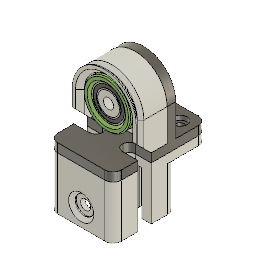
idler-pulley (Autodesk Fusion 360 design; units mm, degrees)
Autodesk Fusion 360 part; units mm, degrees
sketch "Sketch1" plane through (0, 0, 0) normal (0, 0, 1) x (1, 0, 0)
  circle A0 centre (0, 0) radius 7.65
  circle A1 centre (0, 0) radius 10.5
  circle A2 centre (0, 0) radius 9.15
  dimension "d871" = 15.3
  dimension "d873" = 1.5
  dimension "d888" = 0
  dimension "d889" = 0
  dimension "d890" = 0
  dimension "d891" = 0
  dimension "d901" = 21
  constraint coincident A0.centre A1.centre
  constraint concentric A0 A1
  measures "d871" diameter of A0
  measures "d901" diameter of A1
extrude "Extrude1" add sketch "Sketch1" along normal blind 4 contours A1 | A2 makes body 1
sketch "Sketch2" plane through (0, 0, 0) normal (0, 1, 0) x (1, 0, 0)
  line L0 (-10.5, -4) -> (10.5, -4)
  line L1 (-10.5, 0) -> (10.5, 0)
  line L2 (10.5, -4) -> (10.5, -3.5)
  line L3 (10.5, -3.5) -> (9, -2)
  line L4 (9, -2) -> (10.5, -0.5)
  line L5 (10.5, -0.5) -> (10.5, 0)
  line L6 (0, 0) -> (0, -4)
  line L7 (7.65, -4) -> (-7.65, -4)
  line L8 (7.65, -4) -> (7.65, 0)
  line L9 (10.5, -0.5) -> (10.5, -3.5)
  line L10 (9, -2) -> (10.5, -2) construction
  dimension "d882" = 1.5
  dimension "d885" = 0.5
  constraint coincident L0.end L2.start
  constraint perpendicular L0 L2
  constraint coincident L1.end L5.end
  constraint vertical L5
  constraint perpendicular L3 L4
  constraint coincident L6.start origin
  constraint perpendicular L1 L6
  constraint coincident L7.start L8.start
  constraint coincident L1 L8.end
  constraint perpendicular L1 L8
  constraint midpoint L9 L10.end
  constraint horizontal L10
  measures "d882" horizontal distance of L2.end L3.end
  measures "d885" distance of L0.end L2.end
revolve "Revolve1" cut sketch "Sketch2" angle 360 about axis through (0, 0, 0) along (0, 0, 1) contours L3 L4 L9 bodies 1
fillet "Fillet1" radius 1 1 edges at (-8.3909, -3.2545, 2) on bodies 1
ref_plane "WorkPlane1" through (0, 0, 610) normal (0, 0, 1) x (1, 0, 0) in component "top cap"
sketch "Sketch1 (2)" plane through (0, 0, 610) normal (0, 0, 1) x (1, 0, 0) in component "top cap"
  line L0 (14.5, 28.2) -> (-14.5, 28.2)
  line L1 (-14.5, 28.2) -> (-14.5, -14.2)
  line L2 (-14.5, -14.2) -> (14.5, -14.2)
  line L3 (14.5, -14.2) -> (14.5, 28.2)
  line L4 (14.5, 0) -> (-14.5, 0) construction
  circle A0 centre (0, 0) radius 2.5
  arc A1 (3.213, -4.7686) -> (2.0816, -4.3) centre (2.0816, -5.9) ccw
  line L5 (-2.0816, -4.3) -> (2.0816, -4.3)
  arc A2 (-2.0816, -4.3) -> (-3.213, -4.7686) centre (-2.0816, -5.9) ccw
  line L6 (-5.2007, -6.7563) -> (-3.213, -4.7686)
  arc A3 (-5.2007, -6.7563) -> (-5.23, -6.8271) centre (-5.13, -6.8271) ccw
  line L7 (-5.23, -7.7) -> (-5.23, -6.8271)
  arc A4 (-5.23, -7.7) -> (-5.13, -7.8) centre (-5.13, -7.7) ccw
  line L8 (-3.6, -7.8) -> (-5.13, -7.8)
  arc A5 (-2.7, -8.7) -> (-3.6, -7.8) centre (-3.6, -8.7) ccw
  line L9 (-2.7, -9) -> (-2.7, -8.7)
  line L10 (-2.7, 8.7) -> (-2.7, 9)
  arc A6 (-3.6, 7.8) -> (-2.7, 8.7) centre (-3.6, 8.7) ccw
  line L11 (-5.13, 7.8) -> (-3.6, 7.8)
  arc A7 (-5.13, 7.8) -> (-5.23, 7.7) centre (-5.13, 7.7) ccw
  line L12 (-5.23, 6.8271) -> (-5.23, 7.7)
  arc A8 (-5.23, 6.8271) -> (-5.2007, 6.7563) centre (-5.13, 6.8271) ccw
  line L13 (-3.213, 4.7686) -> (-5.2007, 6.7563)
  arc A9 (-3.213, 4.7686) -> (-2.0816, 4.3) centre (-2.0816, 5.9) ccw
  line L14 (2.0816, 4.3) -> (-2.0816, 4.3)
  arc A10 (2.0816, 4.3) -> (3.213, 4.7686) centre (2.0816, 5.9) ccw
  line L15 (5.2007, 6.7563) -> (3.213, 4.7686)
  arc A11 (5.2007, 6.7563) -> (5.23, 6.8271) centre (5.13, 6.8271) ccw
  line L16 (5.23, 7.7) -> (5.23, 6.8271)
  arc A12 (5.23, 7.7) -> (5.13, 7.8) centre (5.13, 7.7) ccw
  line L17 (3.6, 7.8) -> (5.13, 7.8)
  arc A13 (2.7, 8.7) -> (3.6, 7.8) centre (3.6, 8.7) ccw
  line L18 (2.7, 9) -> (2.7, 8.7)
  line L19 (2.7, -8.7) -> (2.7, -9)
  arc A14 (3.6, -7.8) -> (2.7, -8.7) centre (3.6, -8.7) ccw
  line L20 (5.13, -7.8) -> (3.6, -7.8)
  arc A15 (5.13, -7.8) -> (5.23, -7.7) centre (5.13, -7.7) ccw
  line L21 (5.23, -6.8271) -> (5.23, -7.7)
  arc A16 (5.23, -6.8271) -> (5.2007, -6.7563) centre (5.13, -6.8271) ccw
  line L22 (3.213, -4.7686) -> (5.2007, -6.7563)
  line L23 (10.2, 10.2) -> (-10.2, 10.2)
  line L24 (-10.2, 10.2) -> (-10.2, -10.2)
  line L25 (-10.2, -10.2) -> (10.2, -10.2)
  line L26 (10.2, -10.2) -> (10.2, 10.2)
  line L27 (-2.7, -9) -> (-2.7, -10.2)
  line L28 (2.7, -9) -> (2.7, -10.2)
  line L29 (-2.7, 9) -> (-2.7, 10.2)
  line L30 (2.7, 9) -> (2.7, 10.2)
  line L31 (14.5, 3) -> (4.5, 3)
  line L32 (4.5, 3) -> (4.5, -3)
  line L33 (4.5, -3) -> (14.5, -3)
  line L34 (14.5, -3) -> (14.5, 3)
  line L35 (-14.5, 3) -> (-4.5, 3)
  line L36 (-4.5, 3) -> (-4.5, -3)
  line L37 (-4.5, -3) -> (-14.5, -3)
  line L38 (-14.5, -3) -> (-14.5, 3)
  line L39 (14.5, 14.2) -> (-14.5, 14.2)
  dimension "d1200" = 10.2
  dimension "d1201" = 10.2
  dimension "d1202" = 10.2
  dimension "d1203" = 10.2
  dimension "d1227" = 6
  dimension "d1228" = 10
  dimension "d1229" = 10
  dimension "d1230" = 6
  dimension "d1239" = 4
  dimension "d1240" = 14
  dimension "d1241" = 29
  constraint horizontal L0
  constraint vertical L1
  constraint horizontal L2
  constraint vertical L3
  constraint midpoint A0.centre L4
  constraint tangent L21 A16
  constraint tangent A15 L21
  constraint tangent L20 A15
  constraint tangent L17 A13
  constraint tangent L6 A3
  constraint tangent A14 L20
  constraint tangent A4 L8
  constraint tangent A13 L18
  constraint tangent L15 A11
  constraint tangent A10 L15
  constraint tangent L14 A10
  constraint tangent L13 A9
  constraint tangent A8 L13
  constraint tangent L8 A5
  constraint tangent L12 A8
  constraint tangent A9 L14
  constraint tangent L11 A7
  constraint tangent L10 A6
  constraint tangent L5 A2
  constraint tangent A6 L11
  constraint tangent A1 L22
  constraint tangent A12 L17
  constraint tangent L16 A12
  constraint tangent A16 L22
  constraint tangent A11 L16
  constraint tangent A5 L9
  constraint tangent A3 L7
  constraint tangent L19 A14
  constraint tangent A2 L6
  constraint tangent L7 A4
  constraint tangent A7 L12
  constraint tangent A1 L5
  constraint coincident L25 L27.end
  constraint perpendicular L25 L27
  constraint coincident L25 L28.end
  constraint perpendicular L25 L28
  constraint coincident L23 L29.end
  constraint perpendicular L23 L29
  constraint coincident L23 L30.end
  constraint perpendicular L23 L30
  constraint parallel L0 L23
  constraint parallel L1 L24
  constraint parallel L2 L25
  constraint parallel L3 L26
  constraint horizontal L31
  constraint vertical L32
  constraint horizontal L33
  constraint vertical L34
  constraint horizontal L35
  constraint vertical L36
  constraint horizontal L37
  constraint vertical L38
  constraint coincident L3 L39.start
  constraint coincident L1 L39.end
  constraint perpendicular L1 L39
  constraint coincident L1 L4.end
  constraint coincident L3 L4.start
  measures "d1200" distance of A0.centre L26
  measures "d1201" distance of L4 L25
  measures "d1202" distance of A0.centre L24
  measures "d1203" distance of A0.centre L23
  measures "d1227" distance of L31.end L32.end
  measures "d1228" distance of L31.start L31.end
  measures "d1229" distance of L36.end L37.end
  measures "d1230" distance of L35.start L37.end
  measures "d1239" distance of L23 L39
  measures "d1240" distance of L0 L39
  measures "d1241" distance of L1.end L2.end
extrude "Extrude1'" add sketch "Sketch1 (2)" along normal blind 4 separate body contours L0 L1 L3 L39 | L1 L3 L23 L24 L26 L31 L35 L39 | L1 L2 L3 L24 L25 L26 L33 L37 | A1 L5 A2 L6 A3 L7 A4 L8 A5 L9 L10 A6 L11 A7 L12 A8 L13 A9 L14 A10 L15 A11 L16 A12 L17 A13 L18 L19 A14 L20 A15 L21 A16 L22 L23 L24 L25 L26 L27 L28 L29 L30 L31 L32 L33 L35 L36 L37 | L10 A6 L11 A7 L12 A8 L13 A9 L14 A10 L15 A11 L16 A12 L17 A13 L18 L23 L29 L30 | A1 L5 A2 L6 A3 L7 A4 L8 A5 L9 L19 A14 L20 A15 L21 A16 L22 L25 L27 L28 | A0 makes body 2 in component "top cap"
extrude "Extrude2" add sketch "Sketch1 (2)" against normal blind 20 contours L1 L3 L23 L24 L26 L31 L35 L39 | L1 L2 L3 L24 L25 L26 L33 L37 | L10 A6 L11 A7 L12 A8 L13 A9 L14 A10 L15 A11 L16 A12 L17 A13 L18 L23 L29 L30 bodies 2 in component "top cap"
fillet "Fillet1'" radius 1.5 4 edges at (10.2, 10.2, 600) (-10.2, 10.2, 600) (-10.2, -10.2, 600) (10.2, -10.2, 600) on bodies 2 in component "top cap"
fillet "Fillet1'" radius 3.75 6 edges at (-14.5, -14.2, 602) (14.5, -14.2, 602) (-14.5, 28.2, 612) (14.5, 28.2, 612) (-14.5, 14.2, 600) (14.5, 14.2, 600) on bodies 2 in component "top cap"
fillet "Fillet2" radius 3 4 edges at (4.5, -3, 612) (4.5, 3, 612) (-4.5, 3, 612) (-4.5, -3, 612) on bodies 2 in component "top cap"
sketch "Sketch3" plane through (0, 0, 614) normal (0, 0, 1) x (-1, 0, 0) in component "top cap"
  arc A0 (-10.75, 14.2) -> (-14.5, 10.45) centre (-10.75, 10.45) ccw
  line L0 (-14.5, 10.45) -> (-14.5, 3)
  line L1 (-10.75, -28.2) -> (10.75, -28.2)
  line L2 (14.5, -24.45) -> (14.5, -3)
  arc A1 (14.5, 10.45) -> (10.75, 14.2) centre (10.75, 10.45) ccw
  line L3 (10.75, 14.2) -> (-10.75, 14.2)
  line L4 (-14.5, 3) -> (-7.5, 3)
  arc A2 (-7.5, -3) -> (-7.5, 3) centre (-7.5, 0) ccw
  line L5 (-7.5, -3) -> (-14.5, -3)
  line L6 (-14.5, -3) -> (-14.5, -24.45)
  line L7 (14.5, -3) -> (7.5, -3)
  arc A3 (7.5, 3) -> (7.5, -3) centre (7.5, 0) ccw
  line L8 (7.5, 3) -> (14.5, 3)
  line L9 (14.5, 3) -> (14.5, 10.45)
  line L10 (0, -28.2) -> (0, 14.2) construction
  arc A4 (-14.5, -24.45) -> (-10.75, -28.2) centre (-10.75, -24.45) ccw
  arc A5 (10.75, -28.2) -> (14.5, -24.45) centre (10.75, -24.45) ccw
  circle A6 centre (-8.5, -22.2) radius 2.3
  circle A7 centre (8.5, -22.2) radius 2.3
  dimension "d1243" = 4.6
  dimension "d67" = 6
  dimension "d68" = 6
  constraint midpoint L1 L10.start
  constraint midpoint L3 L10.end
  constraint symmetric L10 A6 A7
  measures "d1243" diameter of A6
  measures "d67" distance of L1 A6.centre
  measures "d68" distance of L6 A6.centre
extrude "Extrude4" cut sketch "Sketch3" against normal up to surface (4 mm away) contours A6 | A7 bodies 2 in component "top cap"
sketch "Sketch4" plane through (0, -14.2, 0) normal (0, -1, 0) x (1, 0, 0) in component "top cap"
  line L0 (10.75, 590) -> (10.75, 614)
  line L1 (10.75, 614) -> (-10.75, 614)
  line L2 (-10.75, 614) -> (-10.75, 590)
  line L3 (-10.75, 590) -> (10.75, 590)
  circle A0 centre (0, 598) radius 2.25
  circle A1 centre (0, 598) radius 4.2
  dimension "d1305" = 4.5
  dimension "d1306" = 8.4
  constraint concentric A0 A1
  measures "d1305" diameter of A0
  measures "d1306" diameter of A1
extrude "Extrude7" cut sketch "Sketch4" against normal up to surface (4 mm away) contours A0 bodies 2 in component "top cap"
extrude "Extrude8" cut sketch "Sketch4" against normal blind 2 contours A1 bodies 2 in component "top cap"
chamfer "Chamfer2" distance 1.5 angle 45 1 edges at (-3.9158, -14.2, 599.5188) on bodies 2 in component "top cap"
ref_plane "WorkPlane1" through (0, 0, 612) normal (0, 0, 1) x (1, 0, 0) in component "top adapter"
sketch "Sketch1 (3)" plane through (0, 0, 614) normal (0, 0, 1) x (1, 0, 0) in component "top adapter"
  line L0 (-14.5, 14.2) -> (14.5, 14.2)
  line L1 (14.5, 14.2) -> (14.5, 10.2)
  line L2 (14.5, 10.2) -> (-14.5, 10.2)
  line L3 (-14.5, 10.2) -> (-14.5, 14.2)
  circle A0 centre (8.5, 22.2) radius 2.3
  circle A1 centre (-8.5, 22.2) radius 2.3
  arc A2 (14.5, 24.45) -> (10.75, 28.2) centre (10.75, 24.45) ccw
  line L4 (10.75, 28.2) -> (-10.75, 28.2)
  arc A3 (-10.75, 28.2) -> (-14.5, 24.45) centre (-10.75, 24.45) ccw
  line L5 (-14.5, 24.45) -> (-14.5, 3)
  line L6 (-14.5, 3) -> (-7.5, 3)
  arc A4 (-7.5, -3) -> (-7.5, 3) centre (-7.5, 0) ccw
  line L7 (-7.5, -3) -> (-14.5, -3)
  line L8 (-14.5, -3) -> (-14.5, -10.45)
  arc A5 (-14.5, -10.45) -> (-10.75, -14.2) centre (-10.75, -10.45) ccw
  line L9 (-10.75, -14.2) -> (10.75, -14.2)
  arc A6 (10.75, -14.2) -> (14.5, -10.45) centre (10.75, -10.45) ccw
  line L10 (14.5, -10.45) -> (14.5, -3)
  line L11 (14.5, -3) -> (7.5, -3)
  arc A7 (7.5, 3) -> (7.5, -3) centre (7.5, 0) ccw
  line L12 (7.5, 3) -> (14.5, 3)
  line L13 (14.5, 3) -> (14.5, 24.45)
  line L14 (0, 14.2) -> (0, 28.2) construction
  circle A8 centre (8.5, 22.2) radius 3.1
  circle A9 centre (-8.5, 22.2) radius 3.1
  circle A10 centre (8.5, 22.2) radius 1.75
  circle A11 centre (-8.5, 22.2) radius 1.75
  point P0 (10.75, 24.45)
  point P1 (10.75, 24.45)
  dimension "d1245" = 4
  dimension "d72" = 29
  dimension "d73" = 14
  dimension "d74" = 6.2
  dimension "d75" = 6.2
  dimension "d79" = 3.5
  dimension "d80" = 3.5
  constraint horizontal L0
  constraint vertical L1
  constraint horizontal L2
  constraint vertical L3
  constraint midpoint L0 L14.start
  constraint vertical L14
  constraint midpoint L4 L14.end
  constraint concentric A0 A8
  constraint concentric A1 A9
  constraint concentric A0 A10
  constraint concentric A1 A11
  measures "d1245" distance of L0.end L1.end
  measures "d72" distance of L0.start L0.end
  measures "d73" distance of L14.start L14.end
  measures "d74" diameter of A8
  measures "d75" diameter of A9
  measures "d79" diameter of A10
  measures "d80" diameter of A11
extrude "Extrude1''" add sketch "Sketch1 (3)" along normal blind 4 separate body contours L0 A2 L4 A3 L5 L13 | L0 L1 L2 L3 L5 L13 | L2 L5 L6 A4 L7 L8 A5 L9 A6 L10 L11 A7 L12 L13 | A0 | A1 | A8 | A9 makes body 3 in component "top adapter"
extrude "Extrude2'" add sketch "Sketch1 (3)" along normal blind 29 from surface at 4 contours L0 L1 L2 L3 L5 L13 bodies 3 in component "top adapter"
extrude "Extrude11" cut sketch "Sketch1 (3)" against normal blind 2 from surface at 4 contours A0 | A1 | A8 | A9 | A10 | A11 bodies 3 in component "top adapter"
fillet "Fillet2'" radius 14.5 2 edges at (14.5, 12.2, 647) (-14.5, 12.2, 647) on bodies 3 in component "top adapter"
sketch "Sketch3 (2)" plane through (0, 10.2, 0) normal (0, -1, 0) x (1, 0, 0) in component "top adapter"
  line L0 (14.5, 618) -> (14.5, 632.5)
  circle A0 centre (-10, 632.5) radius 1.75
  line L1 (-10, 632.5) -> (10, 632.5) construction
  circle A1 centre (10, 632.5) radius 1.75
  line L2 (-14.5, 632.5) -> (-14.5, 618)
  line L3 (-14.5, 618) -> (14.5, 618)
  arc A2 (14.5, 632.5) -> (-14.5, 632.5) centre (0, 632.5) ccw
  dimension "d1283" = 3.5
  dimension "d1284" = 3.5
  dimension "d1285" = 20
  constraint coincident A0.centre L1.start
  constraint horizontal L1
  constraint coincident L1.end A1.centre
  measures "d1283" diameter of A0
  measures "d1284" diameter of A1
  measures "d1285" distance of A0.centre L1.end
extrude "Extrude4'" cut sketch "Sketch3 (2)" against normal up to surface (4 mm away) contours A0 | A1 bodies 3 in component "top adapter"
sketch "Sketch3 (3)" plane through (0, 10.2, 0) normal (0, -1, 0) x (1, 0, 0) in component "top idler"
  line L0 (0, 647) -> (0, 618) construction
  circle A0 centre (0, 632.5) radius 4.9
  circle A1 centre (0, 632.5) radius 7
  circle A2 centre (0, 632.5) radius 2.3
  circle A3 centre (-10, 632.5) radius 1.75
  circle A4 centre (10, 632.5) radius 1.75
  arc A5 (14.5, 632.5) -> (-14.5, 632.5) centre (0, 632.5) ccw
  line L1 (-14.5, 632.5) -> (-14.5, 618)
  line L2 (-14.5, 618) -> (14.5, 618)
  line L3 (14.5, 618) -> (14.5, 632.5)
  circle A6 centre (-10, 632.5) radius 2.3
  circle A7 centre (10, 632.5) radius 2.3
  dimension "d1248" = 9.8
  dimension "d1249" = 14
  dimension "d1292" = 0
  dimension "d1293" = 0
  dimension "d1294" = 0
  dimension "d1295" = 0
  dimension "d25" = 0
  dimension "d26" = 0
  dimension "d27" = 0
  dimension "d28" = 0
  dimension "d61" = 4.6
  dimension "d94" = 4.6
  dimension "d95" = 4.6
  constraint midpoint L0 A0.centre
  constraint concentric A0 A1
  constraint concentric A1 A2
  constraint midpoint L0.end L2
  constraint concentric A3 A6
  constraint concentric A4 A7
  measures "d1248" diameter of A0
  measures "d1249" diameter of A1
  measures "d61" diameter of A2
  measures "d94" diameter of A6
  measures "d95" diameter of A7
extrude "Extrude5" add sketch "Sketch3 (3)" along normal blind 4 separate body contours A0 | A1 | A2 | A5 L1 L2 L3 makes body 4 in component "top idler"
extrude "Extrude6" add sketch "Sketch3 (3)" along normal blind 4 from surface at 4 contours A0 | A1 | A2 bodies 4 in component "top idler"
extrude "Extrude7'" add sketch "Sketch3 (3)" along normal blind 4 from surface at 8 contours A0 | A2 bodies 4 in component "top idler"
extrude "Extrude18" cut sketch "Sketch3 (3)" against normal blind 8 from surface at 12 contours A2 bodies 4 in component "top idler"
sketch "Sketch4 (2)" plane through (0, 6.2, 0) normal (0, -1, 0) x (1, 0, 0) in component "top idler"
  circle A0 centre (0, 632.5) radius 7
  circle A1 centre (0, 632.5) radius 14.5
  circle A2 centre (0, 632.5) radius 13
  line L0 (13, 618) -> (13, 632.5)
  line L1 (0, 632.5) -> (14.5, 632.5) construction
  line L2 (0, 632.5) -> (0, 647) construction
  line L3 (-13, 618) -> (-13, 632.5)
  line L4 (14.5, 618) -> (14.5, 632.5)
  arc A3 (14.5, 632.5) -> (-14.5, 632.5) centre (0, 632.5) ccw
  line L5 (-14.5, 632.5) -> (-14.5, 618)
  line L6 (-14.5, 618) -> (14.5, 618)
  circle A4 centre (-10, 632.5) radius 2.3
  circle A5 centre (10, 632.5) radius 2.3
  dimension "d1260" = 29
  dimension "d1261" = 1.5
  dimension "d81" = 1.5
  constraint concentric A0 A1
  constraint coincident A0.centre A1.centre
  constraint coincident A1 L1.end
  constraint coincident L0.end L1
  constraint symmetric L0.start L2 L3.start
  constraint symmetric L0.end L2 L3.end
  constraint coincident L3.start L6
  constraint horizontal L1
  measures "d1260" diameter of A1
  measures "d81" distance of L3 L5
extrude "Extrude8'" add sketch "Sketch4 (2)" along normal blind 10 contours A1 A2 L0 L3 A3 | A1 L0 L4 L6 | A1 L3 L5 L6 bodies 4 in component "top idler"
sketch "Sketch5" plane through (0, 0, 618) normal (0, 0, -1) x (1, 0, 0) in component "top idler"
  line L0 (-13, 3.8) -> (-11, 1.8)
  line L1 (-11, 1.8) -> (-13, -0.2)
  line L2 (-14.5, 3.3) -> (-13, 1.8)
  line L3 (-13, 1.8) -> (-14.5, 0.3)
  line L4 (-13, 1.8) -> (-11, 1.8) construction
  line L5 (-14.5, -10.2) -> (14.5, -10.2)
  line L6 (14.5, -10.2) -> (14.5, 3.8)
  line L7 (14.5, 3.8) -> (13, 3.8)
  line L8 (13, 3.8) -> (13, -6.2)
  line L9 (13, -6.2) -> (-13, -6.2)
  line L10 (-13, -6.2) -> (-13, 3.8)
  line L11 (-13, 3.8) -> (-14.5, 3.8)
  line L12 (-14.5, 3.8) -> (-14.5, -10.2)
  dimension "d1265" = 45
  dimension "d1266" = 45
  dimension "d1267" = 2
  dimension "d1268" = 45
  dimension "d1269" = 45
  dimension "d1270" = 2
  constraint coincident L0.start L10.end
  constraint coincident L1.end L10
  constraint coincident L2.start L12
  constraint coincident L3.end L12
  constraint horizontal L4
  measures "d1265" angle of L0 L10
  measures "d1266" angle of L1 L10
  measures "d1267" distance of L0.end L10
  measures "d1268" angle of L2 L12
  measures "d1269" angle of L3 L12
  measures "d1270" distance of L0.end L2.end
sweep "Sweep1" add profiles "Sketch5" along 3 edges at (-13, -3.8, 625.25) (0, -3.8, 645.5) (13, -3.8, 625.25) section 1 contours L0 L1 L10 on bodies 4 bodies 4 in component "top idler"
sweep "Sweep2" cut profiles "Sketch5" along 3 edges at (14.5, -3.8, 625.25) (0, -3.8, 647) (-14.5, -3.8, 625.25) section 1 contours L2 L3 L12 on bodies 4 bodies 4 in component "top idler"
extrude "Extrude2''" add 1 faces at (9.4824, -0.9017, 4) along direction (0, 0, 1) blind 1 on bodies 1 bodies 1
extrude "Extrude3" add 1 faces at (9.4824, -0.9017, 0) along direction (0, 0, -1) blind 1 on bodies 1 bodies 1
chamfer "Chamfer1" distance 1 angle 45 2 edges at (-7.1323, -2.7664, -1) (-7.1323, 2.7664, 5) on bodies 1
chamfer "Chamfer2'" distance 0.5 angle 45 2 edges at (-9.7894, 3.797, -1) (-9.7894, -3.797, 5) on bodies 1
sketch "Sketch1 (4)" plane through (0, 0, 0) normal (0, 1, 0) x (1, 0, 0) in component "10x15x4mm bearing v1"
  circle A0 centre (0, 0) radius 4.9
  circle A1 centre (0, 0) radius 7.7
  circle A2 centre (0, 0) radius 7.1
  circle A3 centre (0, 0) radius 5.5
  dimension "d1_1" = 9.8
  dimension "d2_1" = 15.4
  dimension "d3_1" = -0.6
  dimension "d4_1" = 0.6
  constraint coincident A0.centre A1.centre
  constraint concentric A0 A1
  measures "d1_1" diameter of A0
  measures "d2_1" diameter of A1
extrude "Extrude1'''" add sketch "Sketch1 (4)" along normal mid plane 4 separate body makes body 5 at (7.6904, 1.3333, 0.3838) makes body 6 at (5.4932, 1.3333, 0.2742) in component "10x15x4mm bearing v1"
extrude "Extrude2'''" add sketch "Sketch1 (4)" along normal mid plane 3.6 separate body contours A2 makes body 7 in component "10x15x4mm bearing v1"
sketch "Sketch12" plane through (-14.5, 0, 0) normal (-1, 0, 0) x (0, -1, 0) in component "top idler"
  line L0 (0.3, 618) -> (0.3, 632.5)
  line L1 (0.3, 632.5) -> (-10.2, 632.5)
  line L2 (-10.2, 632.5) -> (-10.2, 618)
  line L3 (-10.2, 618) -> (0.3, 618)
  line L4 (-3, 614) -> (-3, 618)
  line L5 (3.8, 632.5) -> (3.8, 618)
  line L6 (0.3, 618) -> (3.8, 618)
  line L7 (-3, 618) -> (15.1241, 636.1241)
  dimension "d91" = 45
  constraint coincident L0.start L3.end
  constraint coincident L5.end L6.end
  constraint coincident L4.end L7.start
  measures "d91" angle of L3 L7
extrude "Extrude19" cut sketch "Sketch12" against normal up to surface (29 mm away) contours L0 L3 L7 | L0 L5 L6 L7 bodies 4 in component "top idler"
component "pully" placed x (1, 0, 0) y (0, 1, 0) z (0, 0, 1) at (0, 0, 0) in component "(Unsaved)"
component "top cap" placed x (1, 0, 0) y (0, 1, 0) z (0, 0, 1) at (0, 0, 0) in component "(Unsaved)"
component "top adapter" placed x (1, 0, 0) y (0, 1, 0) z (0, 0, 1) at (0, 0, 0) in component "(Unsaved)"
component "top idler" placed x (1, 0, 0) y (0, 1, 0) z (0, 0, 1) at (0, 0, 0) in component "(Unsaved)"
component "10x15x4mm bearing v1" placed x (1, 0, 0) y (0, 1, 0) z (0, 0, 1) at (0, 0, 0) in component "(Unsaved)"
equation "d901 = pully"
equation "d1243 = M3set"
equation "d1247 = ( 29 / 2 ) * 1 mm"
equation "d1283 = M3hole"
equation "d1284 = M3hole"
equation "d1305 = M4hole"
equation "pully = 21 mm"
equation "M3set = 4.6 mm"
equation "M3hole = 3.5 mm"
equation "M3Head = 6.2 mm"
equation "d74 = M3Head"
equation "d75 = M3Head"
equation "d79 = M3hole"
equation "d80 = M3hole"
equation "d94 = M3set"
equation "d95 = M3set"
equation "M4hole = 4.5 mm"
named bodies: "pully", "idler-coupler", "idler-holder", "idler-mount"
